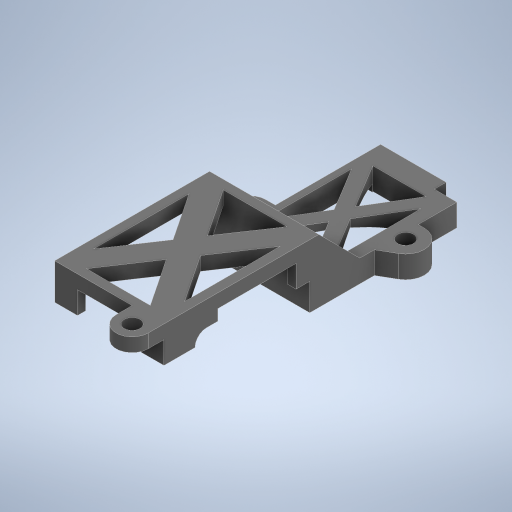
# Autodesk Inventor part: body_under_remake
Saved by Autodesk Inventor 2024.1 (Build 281209000, 209)
## iProperties
Created: 2024-07-01
Part Number: body_under_remake
Material: 一般
Document SubType Name: Modeling
Designer: hibik
Density: 1 g/cm^3
Appearance: 既定
Author: hibik
Autodesk Inventor part; units mm, degrees
ref_plane "YZ Plane" through (0, 0, 0) normal (1, 0, 0) x (0, 1, 0)
ref_plane "XZ Plane" through (0, 0, 0) normal (0, 1, 0) x (-1, 0, 0)
ref_plane "XY Plane" through (0, 0, 0) normal (0, 0, 1) x (1, 0, 0)
sketch "スケッチ1" plane through (0, 0, 0) normal (0, 1, 0) x (-1, 0, 0)
  line L0 (70, 7.5) -> (50, 7.5)
  line L1 (50, 7.5) -> (50, -22.5)
  line L2 (50, -22.5) -> (70, -22.5)
  line L3 (70, -22.5) -> (70, 7.5)
  line L4 (72, 9.5) -> (48, 9.5)
  line L5 (48, 9.5) -> (48, -24.5)
  line L6 (48, -24.5) -> (72, -24.5)
  line L7 (72, -24.5) -> (72, 9.5)
  line L8 (72, 9.5) -> (67, 9.5)
  line L9 (67, 9.5) -> (67, 4.5)
  line L10 (67, 4.5) -> (72, 4.5)
  line L11 (72, 4.5) -> (72, 9.5)
  line L12 (72, -24.5) -> (67, -24.5)
  line L13 (67, -24.5) -> (67, -19.5)
  line L14 (67, -19.5) -> (72, -19.5)
  line L15 (72, -19.5) -> (72, -24.5)
  line L16 (48, 9.5) -> (53, 9.5)
  line L17 (53, 9.5) -> (53, 4.5)
  line L18 (53, 4.5) -> (48, 4.5)
  line L19 (48, 4.5) -> (48, 9.5)
  line L20 (48, -24.5) -> (53, -24.5)
  line L21 (53, -24.5) -> (53, -19.5)
  line L22 (53, -19.5) -> (48, -19.5)
  line L23 (48, -19.5) -> (48, -24.5)
  line L24 (67.5, -27.3) -> (52.5, -27.3)
  line L25 (52.5, -27.3) -> (52.5, -52.3)
  line L26 (52.5, -52.3) -> (67.5, -52.3)
  line L27 (67.5, -52.3) -> (67.5, -27.3)
  line L28 (72, -24.5) -> (48, -24.5)
  line L29 (48, -24.5) -> (48, -53.8)
  line L30 (48, -53.8) -> (72, -53.8)
  line L31 (72, -53.8) -> (72, -24.5)
  line L32 (70, 70) -> (-70, 70)
  line L33 (-70, 70) -> (-70, -70)
  line L34 (-70, -70) -> (70, -70)
  line L35 (70, -70) -> (70, 70)
  line L36 (72, 0) -> (48, 0) construction
  point P0 (0, 0)
  point P1 (72, -7.5)
  point P2 (70, -7.5)
  point P3 (60, -24.5)
  point P4 (60, -22.5)
  point P5 (60, -27.3)
  point P6 (70, 0)
  point P7 (0, 70)
  point P8 (50, -19.5)
  point P9 (48, -19.5)
  point P10 (72, -19.5)
  point P11 (70, -19.5)
  point P12 (67, -22.5)
  point P13 (53, -24.5)
  point P14 (53, -22.5)
  point P15 (48, 4.5)
  point P16 (50, 4.5)
  point P17 (53, 7.5)
  point P18 (53, 9.5)
  point P19 (67, 9.5)
  point P20 (67, 7.5)
  point P21 (70, 4.5)
  point P22 (72, 4.5)
  dimension "d0" = 20
  dimension "d1" = 30
  dimension "d2" = 24
  dimension "d3" = 34
  dimension "d4" = 5
  dimension "d6" = 4.8
  dimension "d7" = 15
  dimension "d8" = 25
  dimension "d9" = 1.5
  dimension "d11" = 7.5
  dimension "d65" = 140
  constraints: 74 end point, 18 parallel, 10 perpendicular, 9 horizontal, 8 equal length, 7 midpoint, 3 point on line, 3 vertical alignment, 2 collinear, 2 horizontal alignment
  measures "d0" distance of L2.end L1.end
  measures "d1" distance of L1.end L0.end
  measures "d2" distance of L4.start L4.end
  measures "d3" distance of L6.end L4.start
  measures "d4" distance of L9.end L10.end
  measures "d6" distance between parallel lines of L24 L2
  measures "d7" distance of L25.end L26.end
  measures "d8" distance of L24.end L25.end
  measures "d9" distance between parallel lines of L30 L26
  measures "d11" distance between parallel lines of L36 L0
  measures "d65" distance of L32.start L32.end
extrude "押し出し1" add sketch "スケッチ1" along normal blind 24 contours L35 L4 L7 L10 L3 | L0 L9 L4 L35 | L0 L1 L18 L5 L4 L17 | L14 L7 L6 L35 L3 | L35 L6 L13 L2 | L1 L2 L21 L6 L5 L22
sketch "スケッチ3" plane through (-70, 0, -22.5) normal (0, 0, 1) x (1, 0, 0)
  circle A0 centre (11.65, 6.5) radius 3.1
  line L0 (20, 0) -> (20, 24) projected
  line L1 (17, 0) -> (20, 0) projected
  circle A1 centre (11.65, 6.5) radius 10
  line L2 (4.15, 13.1144) -> (19.15, 13.1144) construction
  line L3 (19.15, 13.1144) -> (19.15, -0.1144)
  line L4 (19.15, -0.1144) -> (4.15, -0.1144) construction
  line L5 (4.15, -0.1144) -> (4.15, 13.1144)
  line L6 (-2, 13.1144) -> (22, 13.1144)
  line L7 (22, 13.1144) -> (22, -3.5)
  line L8 (22, -3.5) -> (-2, -3.5)
  line L9 (-2, -3.5) -> (-2, 13.1144)
  line L10 (-2, 0) -> (-2, 24) projected
  line L11 (22, 0) -> (22, 24) projected
  line L12 (-2, -3.5) -> (22, -3.5)
  line L13 (22, -3.5) -> (22, -4)
  line L14 (22, -4) -> (-2, -4)
  line L15 (-2, -4) -> (-2, -3.5)
  line L16 (8.55, 13.1144) -> (14.75, 13.1144)
  line L17 (14.75, 13.1144) -> (14.75, 6.5)
  line L18 (14.75, 6.5) -> (8.55, 6.5) construction
  line L19 (8.55, 6.5) -> (8.55, 13.1144)
  line L20 (0, 0) -> (0, 24) projected
  line L21 (4.15, -0.1144) -> (4.15, -4)
  line L22 (19.15, -0.1144) -> (19.15, -4)
  line L23 (0, 18) -> (20, 18)
  line L24 (20, 18) -> (22, 18)
  point P0 (70, 0)
  point P1 (11.65, 13.1144)
  point P2 (20, 0.9975)
  point P3 (19.2493, 0)
  point P4 (14.75, 13.1144)
  point P5 (8.55, 6.5)
  point P6 (20, 5)
  point P7 (19.15, 13.1144)
  point P8 (11.65, -3.5)
  point P9 (4.15, 13.1144)
  point P10 (19.15, -0.1144)
  point P11 (19.15, 13.1144)
  point P12 (19.1, 0)
  point P13 (19.15, -0.1144)
  point P14 (0, 13.1144)
  point P15 (20, 13.1144)
  dimension "d18" = 6.2
  dimension "d20" = 6.5
  dimension "d22" = 20
  dimension "d23" = 15
  dimension "d25" = 0.5
  dimension "d228" = 11.65
  dimension "d272" = 11.5
  constraints: 40 end point, 8 parallel, 8 perpendicular, 6 point on line, 4 collinear, 4 horizontal, 3 midpoint, 2 point on circle, 1 centre point, 1 coincident, 1 tangent, 1 vertical, 1 vertical alignment, 3 other
  measures "d20" distance from line of L1 point (11.65, 6.5)
  measures "d22" diameter of A1
  measures "d23" distance of L2.start L2.end
  measures "d25" distance of L12.end L13.end
  measures "d228" distance from line of point (11.65, 6.5) L20
  measures "d272" distance from line of A1.centre L23
extrude "押し出し2" add sketch "スケッチ3" against normal blind 4.8 contours L6 A1 | A1 L6 L20 L23 L0 | L0 L24 L11 L6
extrude "押し出し3" add sketch "スケッチ3" against normal blind 32.3 contours A1 L6 L20 L23 L0 | L0 L24 L11 L6
sketch "スケッチ48" plane through (-70, 0, -54.8) normal (0, 0, -1) x (-1, 0, 0)
  line L0 (0, 13.1144) -> (0, 18) projected
  line L1 (0, 18) -> (-22, 18) projected
  line L2 (-22, 18) -> (-22, 13.1144) projected
  line L3 (-22, 13.1144) -> (-19.15, 13.1144) projected
  arc A0 (-4.15, 13.1144) -> (-19.15, 13.1144) centre (-11.65, 6.5) ccw projected
  line L4 (-4.15, 13.1144) -> (0, 13.1144) projected
  circle A1 centre (-11.65, 6.5) radius 10
  line L5 (-22.9987, 14.75) -> (-5.9987, 14.75)
  line L6 (-5.9987, 14.75) -> (-5.9987, -1.75)
  line L7 (-5.9987, -1.75) -> (-22.9987, -1.75)
  line L8 (-22.9987, -1.75) -> (-22.9987, 14.75)
  line L9 (-4.15, 13.1144) -> (-5.9987, 13.1144)
  point P0 (-70, 0)
  point P1 (-22, 14.75)
  point P2 (-17.3013, 14.75)
  point P3 (-5.9987, 14.75)
  dimension "d273" = 20
  dimension "d274" = 16.5
  dimension "d275" = 17
  constraints: 10 end point, 2 horizontal, 2 parallel, 2 point on circle, 1 centre point, 1 coincident, 1 perpendicular, 1 point on line
  measures "d273" diameter of A1
  measures "d274" distance of L7.end L5.start
  measures "d275" distance of L6.end L7.end
extrude "押し出し54" add sketch "スケッチ48" along normal blind 1.1 contours L4 A0 L5 L2 L1 L0 | L9 L6 A0
sketch "スケッチ49" plane through (-70, 0, -55.9) normal (0, 0, -1) x (-1, 0, 0)
  line L0 (-22, 18) -> (-22, 14.75) projected
  line L1 (-22, 14.75) -> (-17.3013, 14.75) projected
  arc A0 (-5.9987, 14.75) -> (-17.3013, 14.75) centre (-11.65, 6.5) ccw projected
  line L2 (-5.9987, 14.75) -> (-5.9987, 13.1144) projected
  line L3 (-5.9987, 13.1144) -> (0, 13.1144) projected
  line L4 (0, 13.1144) -> (0, 18) projected
  line L5 (0, 18) -> (-22, 18) projected
  circle A1 centre (-11.65, 6.5) radius 9.2
  line L6 (-5.9987, 13.1144) -> (-5.2555, 13.1144)
  line L7 (-22, 13.95) -> (-17.0479, 13.95)
  line L8 (-22, 13.95) -> (-22, 14.75)
  line L9 (-22, 18) -> (-22, 14.75) projected
  line L10 (-6.7987, 15.2444) -> (-6.7987, 13.1144)
  line L11 (-6.7987, 13.1144) -> (-5.9987, 13.1144)
  point P0 (-70, 0)
  point P1 (-6.7987, 14.3169)
  dimension "d278" = 0.8
  dimension "d279" = 0.8
  dimension "d280" = 0.8
  constraints: 10 end point, 3 point on circle, 2 horizontal, 2 vertical, 1 centre point, 1 coincident, 1 collinear, 1 perpendicular
  measures "d278" radial gap between concentric circles of A0 A1
  measures "d279" distance between parallel lines of L1 L7
  measures "d280" distance between parallel lines of L2 L10
extrude "押し出し55" add sketch "スケッチ49" along normal blind 1.5 contours L5 L4 L3 A1 L2 A0 L1 L0 | L1 A0 L10 A1 L7 L8 | A0 L2 A1 L10 | L3 L2 A1 | A1 L2 L11 L10
sketch "スケッチ50" plane through (0, 0, 0) normal (0, -1, 0) x (1, 0, 0)
  line L0 (-48, 9.5) -> (-48, 4.5) projected
  line L1 (-67, -24.5) -> (-72, -24.5) projected
  line L2 (-48, 9.5) -> (-72, 9.5)
  line L3 (-72, 9.5) -> (-72, -24.5)
  line L4 (-72, -24.5) -> (-48, -24.5)
  line L5 (-48, -24.5) -> (-48, 9.5)
  point P0 (0, 0)
  constraints: 8 end point, 2 parallel, 1 horizontal, 1 perpendicular
extrude "押し出し56" cut sketch "スケッチ50" against normal up to surface (13.1144 mm away)
sketch "スケッチ51" plane through (-53, 13.1144, 9.5) normal (0, -1, 0) x (1, 0, 0)
  line L0 (5, 0) -> (5, -5) projected
  line L1 (5, 0) -> (-19, 0)
  line L2 (-19, 0) -> (-19, -32)
  line L3 (-19, -32) -> (5, -32)
  line L4 (5, -32) -> (5, 0)
  line L5 (-17, -32) -> (3, -32) projected
  line L6 (-19, -34) -> (-19, -29) projected
  point P0 (53, -9.5)
  point P1 (0, -32)
  constraints: 8 end point, 2 collinear, 2 parallel, 1 horizontal, 1 perpendicular
extrude "押し出し57" cut sketch "スケッチ51" against normal blind 5.986
sketch "スケッチ52" plane through (-70, 0, -54.8) normal (0, 0, -1) x (-1, 0, 0)
  arc A0 (-4.15, 13.1144) -> (-19.15, 13.1144) centre (-11.65, 6.5) ccw projected
  line L0 (-19.15, 13.1144) -> (-4.15, 13.1144) projected
  point P0 (-70, 0)
extrude "押し出し58" add sketch "スケッチ52" against normal blind 2.5
sketch "スケッチ53" plane through (0, 24, 0) normal (0, 1, 0) x (1, 0, 0)
  line L0 (-72, -4.5) -> (-72, -9.5) projected
  line L1 (-72, -9.5) -> (-48, -9.5)
  line L2 (-48, -9.5) -> (-48, 24.5)
  line L3 (-48, 24.5) -> (-72, 24.5)
  line L4 (-72, 24.5) -> (-72, -9.5)
  point P0 (0, 0)
  constraints: 8 end point, 2 parallel, 1 coincident, 1 horizontal, 1 perpendicular
sketch "スケッチ54" plane through (-70, 24, -22.5) normal (0, 0, 1) x (1, 0, 0)
  line L0 (3, -6) -> (3, 0) projected
  line L1 (3, 0) -> (17, 0)
  line L2 (17, 0) -> (17, -6)
  line L3 (17, -6) -> (3, -6)
  line L4 (3, -6) -> (3, 0)
  point P0 (70, -24)
  point P1 (3, -6)
  constraints: 8 end point, 2 parallel, 1 coincident, 1 horizontal, 1 perpendicular
extrude "押し出し59" add sketch "スケッチ54" against normal up to surface (2 mm away)
extrude "押し出し60" add sketch "スケッチ53" along normal blind 3
chamfer "面取り4" distance 9 angle 45 1 edges at (-59, 18, -24.5)
sketch "スケッチ55" plane through (-72, 13.1144, -22.5) normal (0, -1, 0) x (1, 0, 0)
  line L0 (2, -2) -> (2, -34.9) projected
  line L1 (2, -34.9) -> (4.65, -34.9)
  line L2 (4.65, -34.9) -> (4.65, -2)
  line L3 (4.65, -2) -> (2, -2)
  line L4 (2, -2) -> (2, -34.9)
  line L5 (2, -2) -> (0, -2) projected
  line L6 (6.15, -4.8) -> (6.15, -29.8) projected
  point P0 (72, 22.5)
  point P1 (2, -2)
  dimension "d296" = 1.5
  constraints: 8 end point, 2 parallel, 1 collinear, 1 horizontal, 1 perpendicular
  measures "d296" distance between parallel lines of L2 L6
extrude "押し出し61" cut sketch "スケッチ55" against normal up to surface (13.8856 mm away)
sketch "スケッチ56" plane through (-48, 18, -33.5) normal (0, 1, 0) x (1, 0, 0)
  line L0 (1.35, 12.8) -> (-2.7012, 12.8)
  line L1 (-7.2, -6.3) -> (-2.7, -6.3) projected
  line L2 (-7.2, -11.1) -> (-7.2, -6.3) projected
  line L3 (0, -11.1) -> (-7.2, -11.1) projected
  line L4 (0, -11.1) -> (0, 3.194) projected
  line L5 (0, 3.194) -> (3.3939, 5.1458)
  arc A0 (3.3939, 5.1458) -> (1.35, 12.8) centre (1.35, 8.7) ccw
  circle A1 centre (1.35, 8.7) radius 1.35
  circle A2 centre (-21.45, -2.7) radius 1.35
  line L6 (-17.9, -6.3) -> (-13.4, -6.3) projected
  line L7 (-17.9, -6.3) -> (-17.9, 18.9) projected
  line L8 (-17.9, 18.9) -> (-15.4, 18.9) projected
  line L9 (-15.4, 18.9) -> (-15.4, 21.2) projected
  line L10 (-16.2013, 21.2) -> (-15.4, 21.2) projected
  line L11 (-15.1513, 22.3) -> (-15.1513, 23.8) projected
  line L12 (-19.3, 23.8) -> (-15.1513, 23.8) projected
  line L13 (-19.3, 23.8) -> (-19.2999, 0.8)
  line L14 (-19.2999, 0.8) -> (-21.45, 0.8)
  arc A3 (-21.45, 0.8) -> (-24.7816, -3.7727) centre (-21.45, -2.7) ccw
  line L15 (-24.7816, -3.7727) -> (-24, -6.2)
  line L16 (-24, -11.1) -> (-24, -6.2)
  line L17 (-13.4, -11.1) -> (-24, -11.1) projected
  line L18 (-13.4, -11.1) -> (-13.4, -6.3) projected
  line L19 (-19.35, 23.9) -> (-19.35, 0) projected
  line L20 (0, 0) -> (0, 23.9) projected
  line L21 (-19.35, 23.9) -> (0, 23.9) projected
  line L22 (-19.35, 0) -> (-19.35, -9) projected
  line L23 (0, -9) -> (0, 0) projected
  line L24 (0, 0) -> (-19.35, 0) projected
  line L25 (-24, -9) -> (-24, -43) projected
  line L26 (-24, -43) -> (0, -43) projected
  line L27 (0, -43) -> (0, -9) projected
  line L28 (0, -9) -> (-19.35, -9) projected
  line L29 (0, -9) -> (-19.35, -9) projected
  line L30 (-16.2013, 21.2) -> (-16.2013, 22.3) projected
  line L31 (-16.2013, 22.3) -> (-15.1513, 22.3) projected
  line L32 (-19.35, -9) -> (-24, -9) projected
  line L33 (0, 0) -> (-19.35, 0) projected
  arc A4 (5.3618, 9.5458) -> (1.35, 12.8) centre (1.35, 8.7) ccw projected
  line L34 (0, 3.1863) -> (5.3618, 9.5458)
  circle A5 centre (1.35, 8.7) radius 1.35 projected
  line L35 (1.35, 12.8) -> (-2.75, 12.8) projected
  line L36 (-19.35, 0.8) -> (-21.45, 0.8) projected
  arc A6 (-21.45, 0.8) -> (-24.7816, -3.7727) centre (-21.45, -2.7) ccw projected
  line L37 (-24.7816, -3.7727) -> (-24, -6.2) projected
  line L38 (-24, -11) -> (-24, -6.2) projected
  circle A7 centre (-21.45, -2.7) radius 1.35 projected
  circle A8 centre (1.35, 8.7) radius 4.1
  point P0 (48, -33.5)
  point P1 (-15.9513, 22.3)
  point P2 (-19.35, 0.8)
  point P3 (0, 12.8)
  point P4 (0, 8.7)
  point P5 (0, 3.194)
  point P6 (-19.3, 0.7)
  point P7 (-15.1513, 23.8)
  point P8 (-13.4, -9)
  point P9 (-17.9, 0)
  point P10 (0, -9.1)
  constraints: 14 end point, 8 concentric, 4 centre point, 4 collinear, 4 point on circle, 1 coincident, 5 other
extrude "押し出し62" add sketch "スケッチ56" against normal up to surface (4.8856 mm away) contours A8 L20 L0 | A0 L34 A8 L20 | A0 A8 L34 | A8 L5 L34 | L34 L5 L20 A8 | L19 L22 L32 L16 L15 A3 L14
sketch "スケッチ57" plane through (0, 27, 0) normal (0, 1, 0) x (1, 0, 0)
  arc A0 (-51.5, -9.5) -> (-55, -13) centre (-51.5, -13) ccw projected
  line L0 (-51.5, -9.5) -> (-55, -9.5) projected
  line L1 (-55, -9.5) -> (-55, -13) projected
  circle A1 centre (-51.5, -13) radius 3.5 projected
  circle A2 centre (-51.5, -13) radius 1.35 projected
  arc A3 (-48, -13) -> (-51.5, -9.5) centre (-51.5, -13) ccw projected
  line L2 (-48, -13) -> (-48, -9.5) projected
  line L3 (-48, -9.5) -> (-51.5, -9.5) projected
  point P0 (0, 0)
extrude "押し出し63" add sketch "スケッチ57" against normal up to surface (3 mm away)
sketch "スケッチ58" plane through (-48, 13.1144, -22.5) normal (1, 0, 0) x (0, 0, -1)
  arc A0 (-20.2, 3.4856) -> (-20.2, 8.4856) centre (-20.2, 5.9856) ccw projected
  line L0 (-22.7, 8.4856) -> (-20.2, 8.4856) projected
  arc A1 (-22.7, 8.4856) -> (-22.7, 3.4856) centre (-22.7, 5.9856) ccw projected
  line L1 (-20.2, 3.4856) -> (-22.7, 3.4856) projected
  line L2 (-32, 5.986) -> (-27, 5.986) projected
  line L3 (-27, 10.8856) -> (-3, 10.8856) projected
  line L4 (-27, 5.986) -> (-20.2, 5.986)
  line L5 (-20.2, 5.986) -> (-20.2, 10.8856)
  line L6 (-20.2, 10.8856) -> (-27, 10.8856)
  line L7 (-27, 10.8856) -> (-27, 5.986)
  point P0 (-22.5, -13.1144)
  point P1 (-25.2, 5.986)
  constraints: 8 end point, 2 parallel, 2 point on line, 1 horizontal, 1 perpendicular
extrude "押し出し64" add sketch "スケッチ58" against normal up to surface (2 mm away) contours L0 A1 L4 L7 L3 L5
sketch "スケッチ59" plane through (-72, 13.1144, -22.5) normal (-1, 0, 0) x (0, 0, 1)
  circle A0 centre (22.7, 5.9856) radius 1.25 projected
  arc A1 (20.2, 8.4856) -> (20.2, 3.4856) centre (20.2, 5.9856) ccw projected
  line L0 (20.2, 3.4856) -> (22.7, 3.4856) projected
  arc A2 (22.7, 3.4856) -> (22.7, 8.4856) centre (22.7, 5.9856) ccw projected
  line L1 (22.7, 8.4856) -> (20.2, 8.4856) projected
  line L2 (27, 5.986) -> (27, 10.8856) projected
  line L3 (20.2, 8.4856) -> (20.2, 10.8856) projected
  line L4 (27, 5.986) -> (20.2, 5.986)
  line L5 (20.2, 5.986) -> (20.2, 10.8856)
  line L6 (20.2, 10.8856) -> (27, 10.8856)
  line L7 (27, 10.8856) -> (27, 5.986)
  point P0 (22.5, -13.1144)
  point P1 (27, 10.8856)
  point P2 (25.2, 5.986)
  constraints: 8 end point, 2 parallel, 1 horizontal, 1 perpendicular
extrude "押し出し65" add sketch "スケッチ59" against normal up to surface (2 mm away) contours A2 L1 L3 L6 L2 L4
sketch "スケッチ60" plane through (0, 27, 0) normal (0, 1, 0) x (1, 0, 0)
  circle A0 centre (-51.5, -13) radius 1.35 projected
  circle A1 centre (-69.45, 30.8) radius 1.35 projected
  circle A2 centre (-46.65, 42.2) radius 1.35 projected
  circle A3 centre (-51.5, -13) radius 1.75
  circle A4 centre (-69.45, 30.8) radius 1.75
  circle A5 centre (-46.65, 42.2) radius 1.75
  point P0 (0, 0)
  dimension "d307" = 3.5
  dimension "d308" = 3.5
  dimension "d309" = 3.5
  constraints: 3 centre point, 3 coincident
  measures "d307" diameter of A3
  measures "d308" diameter of A4
  measures "d309" diameter of A5
extrude "押し出し66" cut sketch "スケッチ60" against normal through all contours A0 | A1 | A2 | A3 | A4 | A5
sketch "スケッチ61" plane through (0, 27, 0) normal (0, 1, 0) x (1, 0, 0)
  circle A0 centre (-51.5, -13) radius 1.35 projected
  line L0 (-55, -9.5) -> (-55, -13) projected
  line L1 (-72, -9.5) -> (-55, -9.5) projected
  line L2 (-72, 27.3) -> (-72, -9.5) projected
  line L3 (-72, 27.3) -> (-67.3, 27.3) projected
  line L4 (-67.3, 27.3) -> (-67.3, 57.4) projected
  line L5 (-48, 57.4) -> (-67.3, 57.4) projected
  line L6 (-48, -13) -> (-48, 57.4) projected
  arc A1 (-55, -13) -> (-48, -13) centre (-51.5, -13) ccw projected
  line L7 (-53.0046, -7.5) -> (-60, 2.9931) projected
  line L8 (-60, 2.9931) -> (-66.9954, -7.5) projected
  line L9 (-66.9954, -7.5) -> (-53.0046, -7.5) projected
  line L10 (-50, -2.9931) -> (-50, 17.9931) projected
  line L11 (-50, 17.9931) -> (-56.9954, 7.5) projected
  line L12 (-56.9954, 7.5) -> (-50, -2.9931) projected
  line L13 (-70, 17.9931) -> (-70, -2.9931) projected
  line L14 (-70, -2.9931) -> (-63.0046, 7.5) projected
  line L15 (-63.0046, 7.5) -> (-70, 17.9931) projected
  line L16 (-66.9954, 22.5) -> (-60, 12.0069) projected
  line L17 (-60, 12.0069) -> (-53.0046, 22.5) projected
  line L18 (-53.0046, 22.5) -> (-66.9954, 22.5) projected
  line L19 (-50.7, 27.3) -> (-65.9, 27.3) projected
  line L20 (-50.7, 27.3) -> (-50.7, 52.5) projected
  line L21 (-50.7, 52.5) -> (-65.9, 52.5) projected
  line L22 (-65.9, 52.5) -> (-65.9, 27.3) projected
  line L23 (-51.9844, 26.5253) -> (-67.1844, 51.7253)
  line L24 (-67.1844, 51.7253) -> (-64.6156, 53.2747)
  line L25 (-64.6156, 53.2747) -> (-49.4156, 28.0747)
  line L26 (-49.4156, 28.0747) -> (-51.9844, 26.5253)
  line L27 (-51.9844, 26.5253) -> (-64.6156, 53.2747) construction
  line L28 (-67.1844, 51.7253) -> (-49.4156, 28.0747) construction
  line L29 (-67.1844, 28.0747) -> (-51.9844, 53.2747)
  line L30 (-51.9844, 53.2747) -> (-49.4156, 51.7253)
  line L31 (-49.4156, 51.7253) -> (-64.6156, 26.5253)
  line L32 (-64.6156, 26.5253) -> (-67.1844, 28.0747)
  line L33 (-67.1844, 28.0747) -> (-49.4156, 51.7253) construction
  line L34 (-51.9844, 53.2747) -> (-64.6156, 26.5253) construction
  point P0 (0, 0)
  point P1 (-58.3, 39.9)
  point P2 (-58.3, 39.9)
  point P3 (-50.7, 49.5958)
  point P4 (-56.5483, 39.9)
  point P5 (-50.7, 30.2042)
  point P6 (-58.3, 42.8042)
  point P7 (-52.4517, 52.5)
  point P8 (-64.1483, 52.5)
  point P9 (-65.9, 30.2042)
  point P10 (-60.0517, 39.9)
  point P11 (-65.9, 49.5958)
  point P12 (-58.3, 36.9958)
  point P13 (-64.1483, 27.3)
  point P14 (-52.4517, 27.3)
  dimension "d312" = 3
  constraints: 24 end point, 8 midpoint, 4 parallel, 2 perpendicular, 1 equal length
  measures "d312" distance between parallel lines of L29 L31
extrude "押し出し67" cut sketch "スケッチ61" against normal through all contours L9 L8 L7 | L12 L11 L10 | L15 L14 L13 | L18 L17 L16 | L19 L31 L23 | L25 L31 L20 | L29 L22 L23 | L25 L21 L29
sketch "スケッチ62" plane through (-67.35, 18, -57.4) normal (0, 1, 0) x (1, 0, 0)
  circle A0 centre (-2.1, -26.6) radius 1.75 projected
  circle A1 centre (-2.1, -26.6) radius 2.75
  point P0 (67.35, -57.4)
  dimension "d315" = 5.5
  constraints: 1 centre point, 1 coincident
  measures "d315" diameter of A1
extrude "押し出し68" cut sketch "スケッチ62" along normal through all contours A0 | A1
sketch "スケッチ63" plane through (-53, 19.1004, 9.5) normal (0, -1, 0) x (1, 0, 0)
  line L0 (3.1, -1.8) -> (-17.1, -1.8)
  line L1 (-17.1, -1.8) -> (-17.1, -32)
  line L2 (-17.1, -32) -> (3.1, -32)
  line L3 (3.1, -32) -> (3.1, -1.8)
  line L4 (5, -32) -> (-19, -32) projected
  line L5 (3, -11.8) -> (3, -27.4931) projected
  line L6 (-17, -27.4931) -> (-17, -11.8) projected
  line L7 (-13.9954, -2) -> (-0.0046, -2) projected
  point P0 (53, -9.5)
  point P1 (-13.9954, -32)
  dimension "d318" = 0.1
  dimension "d319" = 0.1
  dimension "d320" = 0.2
  constraints: 8 end point, 2 parallel, 1 collinear, 1 horizontal, 1 perpendicular
  measures "d318" distance between parallel lines of L3 L5
  measures "d319" distance between parallel lines of L1 L6
  measures "d320" distance between parallel lines of L0 L7
extrude "押し出し69" cut sketch "スケッチ63" against normal up to surface (4.8996 mm away)
sketch "スケッチ64" plane through (-70, 0, -54.8) normal (0, 0, -1) x (-1, 0, 0)
  line L0 (-17.3013, 14.75) -> (-22, 14.75) projected
  line L1 (-22, 14.75) -> (-22, 13.1144) projected
  line L2 (-22, 13.1144) -> (-5.9987, 13.1144) projected
  line L3 (-5.9987, 14.75) -> (-5.9987, 13.1144) projected
  arc A0 (-5.9987, 14.75) -> (-17.3013, 14.75) centre (-11.65, 6.5) ccw projected
  circle A1 centre (-11.65, 6.5) radius 10.25
  line L4 (-22, 14.75) -> (-17.3782, 14.75)
  line L5 (-17.3782, 14.75) -> (-17.3782, 15)
  line L6 (-17.3782, 15) -> (-22, 15)
  line L7 (-22, 15) -> (-22, 14.75)
  line L8 (-5.9987, 13.1144) -> (-5.7487, 13.1144)
  line L9 (-5.7487, 13.1144) -> (-5.7487, 14.8807)
  line L10 (-5.7487, 14.8807) -> (-5.9987, 14.8807)
  line L11 (-5.9987, 14.8807) -> (-5.9987, 13.1144)
  point P0 (-70, 0)
  dimension "d323" = 20.5
  dimension "d324" = 0.25
  dimension "d325" = 0.25
  constraints: 16 end point, 4 parallel, 2 horizontal, 2 perpendicular, 2 point on circle, 1 centre point, 1 coincident
  measures "d323" diameter of A1
  measures "d324" distance of L6.end L0.end
  measures "d325" distance of L2.end L8.end
extrude "押し出し70" cut sketch "スケッチ64" along normal blind 1.1 contours A0 L3 L2 A1 L0 | L0 L5 A1 L10 L11 A0 | L0 A1 L5 | L11 L10 L9 L8 L3 | A1 L2 L1 L0 | L0 L7 L6 A1
sketch "スケッチ65" plane through (-52.9521, 13.95, -55.9) normal (0, -1, 0) x (1, 0, 0)
  line L0 (4.9521, 0) -> (0, 0) projected
  line L1 (0, 0) -> (0, -1.5) projected
  line L2 (4.9521, -1.5) -> (0, -1.5) projected
  line L3 (4.9521, 0) -> (4.9521, -1.5) projected
  line L4 (4.9521, 0) -> (0, 0) projected
  line L5 (0, 0) -> (0, 1.1)
  line L6 (-11.2992, 1.1) -> (0.3303, 1.1) projected
  line L7 (0, 1.1) -> (4.9521, 1.1)
  line L8 (4.9521, 1.1) -> (4.9521, 0)
  point P0 (52.9521, 55.9)
  point P1 (0, 1.1)
  constraints: 6 end point, 2 perpendicular, 1 coincident
extrude "押し出し71" cut sketch "スケッチ65" against normal through all
